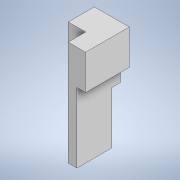
# Autodesk Inventor part: Součást3
Saved by Autodesk Inventor 2022 (Build 260153000, 153)
## iProperties
Created: 2022-03-14
Part Number: Součást3
Material: Všeobecné
Document SubType Name: Modeling
Designer: Šimon
Density: 1 g/cm^3
Appearance: Výchozí
Author: Šimon
Autodesk Inventor part; units mm, degrees
ref_plane "YZ Plane" through (0, 0, 0) normal (1, 0, 0) x (0, 1, 0)
ref_plane "XZ Plane" through (0, 0, 0) normal (0, 1, 0) x (-1, 0, 0)
ref_plane "XY Plane" through (0, 0, 0) normal (0, 0, 1) x (1, 0, 0)
sketch "Náčrt1" plane through (0, 0, 0) normal (0, 0, 1) x (1, 0, 0)
  line L0 (0, 0) -> (20, 0)
  line L1 (20, 0) -> (20, 60)
  line L2 (20, 60) -> (0, 60)
  line L3 (0, 60) -> (0, 0)
  dimension "d0" = 20
  dimension "d1" = 60
  constraints: 8 end point, 2 parallel, 1 horizontal, 1 perpendicular
  measures "d0" distance of L2.end L1.end
  measures "d1" distance of L1.end L0.end
extrude "Vysunutí1" add sketch "Náčrt1" along normal blind 25
sketch "Náčrt2" plane through (0, 0, 25) normal (0, 0, 1) x (1, 0, 0)
  line L0 (20, 60) -> (0, 60) projected
  line L1 (0, 0) -> (20, 0) projected
  line L2 (0, 60) -> (10, 60)
  line L3 (10, 60) -> (10, 0)
  line L4 (10, 0) -> (0, 0)
  line L5 (0, 0) -> (0, 60)
  dimension "d4" = 10
  constraints: 8 end point, 2 parallel, 1 horizontal, 1 midpoint, 1 perpendicular
  measures "d4" distance of L3.end L4.end
extrude "Vysunutí2" cut sketch "Náčrt2" against normal blind 10
sketch "Náčrt3" plane through (0, 0, 0) normal (-1, 0, 0) x (0, 0, 1)
  line L0 (0, 0) -> (25, 0) projected
  line L1 (0, 0) -> (5, 0)
  line L2 (5, 0) -> (5, 30)
  line L3 (5, 30) -> (0, 30)
  line L4 (0, 30) -> (0, 0)
  dimension "d7" = 5
  dimension "d8" = 30
  constraints: 8 end point, 2 parallel, 1 horizontal, 1 perpendicular
  measures "d7" distance of L3.end L2.end
  measures "d8" distance of L2.end L1.end
extrude "Vysunutí3" cut sketch "Náčrt3" against normal through all
sketch "Náčrt4" plane through (0, 0, 25) normal (0, 0, 1) x (1, 0, 0)
  line L0 (20, 0) -> (20, 60) projected
  line L1 (20, 0) -> (15, 0)
  line L2 (15, 0) -> (15, 40)
  line L3 (15, 40) -> (20, 40)
  line L4 (20, 40) -> (20, 0)
  point P0 (0, 0)
  dimension "d11" = 5
  dimension "d12" = 40
  constraints: 8 end point, 2 parallel, 1 horizontal, 1 perpendicular
  measures "d11" distance of L2.end L3.end
  measures "d12" distance of L1.end L2.end
extrude "Vysunutí4" cut sketch "Náčrt4" against normal through all
